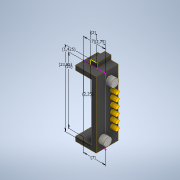
# Autodesk Inventor part: fast_battery
Saved by Autodesk Inventor 2020 (Build 240168000, 168)
## iProperties
Created: 2022-07-18
Part Number: fast_battery
Material: Типовые
Document SubType Name: Modeling
Designer: akapu
Density: 1 g/cm^3
Appearance: По умолчанию
Author: akapu
Autodesk Inventor part; units mm, degrees
ref_plane "YZ Plane" through (0, 0, 0) normal (1, 0, 0) x (0, 1, 0)
ref_plane "XZ Plane" through (0, 0, 0) normal (0, 1, 0) x (-1, 0, 0)
ref_plane "XY Plane" through (0, 0, 0) normal (0, 0, 1) x (1, 0, 0)
sketch "Эскиз1" plane through (0, 0, 0) normal (0, 1, 0) x (-1, 0, 0)
  line L0 (0, -6.5) -> (-2.25, -6.5)
  line L1 (-2.25, -6.5) -> (-4.25, -6.5)
  line L2 (-2.25, -6.5) -> (-4.25, -6.5)
  line L3 (-6.5, -6.5) -> (-4.25, -6.5)
  line L4 (0, -6.5) -> (0, 0.5)
  line L5 (0, 0.5) -> (-6.5, 0.5)
  line L6 (-6.5, 0.5) -> (-6.5, -6.5)
  line L7 (-2.25, -6.5) -> (-2.25, -1.5)
  line L8 (-2.25, -1.5) -> (-4.25, -1.5)
  line L9 (-4.25, -1.5) -> (-4.25, -6.5)
  point P0 (0, 0)
  dimension "d2" = 2.25
  dimension "d4" = 2
  dimension "d31" = 7
  dimension "d32" = 5
  constraints: 20 end point, 4 perpendicular, 2 vertical, 1 horizontal
  measures "d2" distance of L0.start L0.end
  measures "d4" distance of L0.end L1.end
  measures "d31" distance of L0.start L4.end
  measures "d32" distance of L0.end L7.end
extrude "Выдавливание1" add sketch "Эскиз1" along normal blind 21
sketch "Эскиз2" plane through (0, 21, 0) normal (0, 1, 0) x (1, 0, 0)
  line L0 (4.25, 2) -> (2.25, 2) projected
  line L1 (4.25, 6.5) -> (2.25, 6.5)
  line L2 (2.25, 6.5) -> (2.25, 2)
  line L3 (2.25, 2) -> (4.25, 2)
  line L4 (4.25, 2) -> (4.25, 6.5)
  point P0 (0, 0)
  constraints: 8 end point, 2 parallel, 1 horizontal, 1 perpendicular
extrude "Выдавливание2" add sketch "Эскиз2" along normal blind 1.425 and the other way blind 22.425
sketch "Эскиз4" plane through (2.25, 0, -2) normal (0, 0, 1) x (1, 0, 0)
  line L0 (0, 22.425) -> (2, 22.425) projected
  line L1 (2, -1.425) -> (0, -1.425) projected
  line L2 (-2.25, 21) -> (4.75, 21) projected
  line L3 (-2.25, 0) -> (4.75, 0) projected
  line L4 (4.75, 0) -> (4.75, 21) projected
  line L5 (-2.25, 1) -> (-2.25, 20) projected
  line L6 (0, 22.425) -> (0, 21) projected
  line L7 (2, 21) -> (2, 22.425) projected
  dimension "d17" = 23.85
  dimension "d18" = 21
  dimension "d19" = 7
  dimension "d20" = 2.25
  dimension "d21" = 2
  dimension "d22" = 2.75
  dimension "d23" = 1.425
  dimension "d24" = 7
  measures "d17" distance between parallel lines of L0 L1
  measures "d18" distance between parallel lines of L2 L3
  measures "d19" distance between parallel lines of L4 L5
  measures "d20" distance between parallel lines of L6 L5
  measures "d21" distance of L0.start L0.end
  measures "d22" distance between parallel lines of L4 L7
  measures "d23" distance of L6.end L0.start
  measures "d24" distance of L3.start L3.end
sketch "Эскиз6" plane through (0, 0, 0.5) normal (0, 0, 1) x (1, 0, 0)
  line L0 (0, 0) -> (0, 1.5)
  line L1 (0, 0) -> (0, 21) projected
  line L2 (0, 21) -> (6.5, 21) projected
  line L3 (0, 21) -> (0, 19.5)
  line L4 (0, 19.5) -> (5, 19.5)
  line L5 (5, 19.5) -> (5, 1.5)
  line L6 (5, 1.5) -> (0, 1.5)
  line L7 (0, 1.5) -> (0, 19.5)
  dimension "d33" = 1.5
  dimension "d34" = 1.5
  dimension "d35" = 5
  constraints: 12 end point, 3 perpendicular, 2 point on line, 1 collinear
  measures "d33" distance of L0.start L0.end
  measures "d34" distance of L1.end L3.end
  measures "d35" distance of L3.end L4.end
extrude "Выдавливание5" cut sketch "Эскиз6" against normal blind 5
sketch "Эскиз7" plane through (6.5, 0, 0.5) normal (1, 0, 0) x (0, 0, -1)
  line L0 (7, 0) -> (7, 21) projected
  line L1 (7, 10.5) -> (7, 18)
  line L2 (7, 18) -> (7, 3)
  line L3 (0, 19.5) -> (0, 1.5) projected
  line L4 (0, 3) -> (7, 3)
  line L5 (0, 18) -> (7, 18)
  line L6 (7, 18) -> (4, 18)
  line L7 (4.5, 18) -> (4.5, 3)
  line L8 (4.5, 3) -> (2, 3)
  circle A0 centre (2, 3) radius 1.25
  circle A1 centre (4.25, 18) radius 1.25
  line L9 (5, 19.5) -> (5, 1.5) projected
  line L10 (5, 1.5) -> (5, 19.5) projected
  line L11 (5, 3) -> (5, 5)
  line L12 (5, 5) -> (5, 7)
  line L13 (5, 7) -> (5, 9)
  line L14 (5, 9) -> (5, 11)
  line L15 (5, 11) -> (5, 13)
  line L16 (5, 13) -> (5, 15)
  circle A2 centre (5, 5) radius 0.6
  circle A3 centre (5, 7) radius 0.6
  circle A4 centre (5, 9) radius 0.6
  circle A5 centre (5, 11) radius 0.6
  circle A6 centre (5, 13) radius 0.6
  circle A7 centre (5, 15) radius 0.6
  point P0 (0.5, 0)
  dimension "d38" = 7.5
  dimension "d39" = 15
  dimension "d40" = 3
  dimension "d41" = 0.5
  dimension "d42" = 2.5
  dimension "d43" = 2.5
  dimension "d44" = 2.5
  dimension "d61" = 2
  dimension "d62" = 2
  dimension "d63" = 2
  dimension "d64" = 2
  dimension "d65" = 2
  dimension "d66" = 2
  dimension "d68" = 1.2
  dimension "d69" = 1.2
  dimension "d70" = 1.2
  dimension "d71" = 1.2
  dimension "d72" = 1.2
  dimension "d73" = 1.2
  constraints: 26 end point, 8 centre point, 8 point on line, 7 coincident, 2 perpendicular, 1 midpoint, 1 parallel, 8 other
  measures "d38" distance of L1.start L1.end
  measures "d39" distance of L1.end L2.end
  measures "d40" distance of L1.end L6.end
  measures "d41" distance of L6.end L7.start
  measures "d42" distance of L7.end L8.end
  measures "d43" diameter of A0
  measures "d44" diameter of A1
  measures "d61" distance of L11.start L11.end
  measures "d62" distance of L11.end L12.end
  measures "d63" distance of L12.end L13.end
  measures "d64" distance of L13.end L14.end
  measures "d65" distance of L14.end L15.end
  measures "d66" distance of L15.end L16.end
  measures "d68" diameter of A2
  measures "d69" diameter of A3
  measures "d70" diameter of A4
  measures "d71" diameter of A5
  measures "d72" diameter of A6
  measures "d73" diameter of A7
extrude "Выдавливание6" add sketch "Эскиз7" along normal blind 1.7 contours A2 L7 L9 | L9 A2 | A1 L9 L5 | L5 L9 A1 | A0 L4 | L4 A0 | A2 L7 | L9 A1 L7 L5 | L5 A1 L9 | L7 A1 L5 | A7 L9 | L9 A7 L7 | A3 L7 | L7 A3 L9 | L9 A3 | L7 A7 | A4 L7 | L7 A4 L9 | A6 L9 L7 | L7 A6 | A6 L9 | L9 A4 | A5 L7 | L7 A5 L9 | L9 A5
